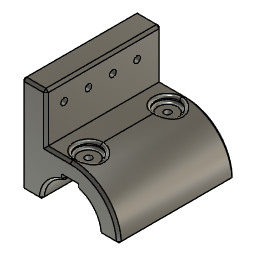
Assembly (Autodesk Fusion 360 archive; units mm, degrees)
design "motorbottlemount"
Autodesk Fusion 360 part; units mm, degrees
sketch "Sketch1" plane through (0, 0, 0) normal (0, 0, 1) x (1, 0, 0)
  line L0 (0, 0) -> (0, 65) construction
  circle A0 centre (0, 0) radius 2.7
  circle A1 centre (0, 65) radius 2.7
  dimension "d1" = 65
  dimension "d2" = 5.4
  dimension "d3" = 5.4
  constraint coincident L0.start A0.centre
  constraint vertical L0
  constraint coincident L0.end A1.centre
  measures "d1" distance of L0.start L0.end
  measures "d2" diameter of A0
  measures "d3" diameter of A1
sketch "Sketch2" plane through (0, 0, 0) normal (0, 1, 0) x (1, 0, 0)
  circle A0 centre (0, 0) radius 23.5
  circle A1 centre (0, 0) radius 40
  line L0 (-40, 0) -> (-40, -80)
  line L1 (-40, -80) -> (0, -80)
  line L2 (0, 0) -> (0, -80)
  line L3 (0, -80) -> (-20, -80)
  line L4 (-20, -80) -> (-20, -40)
  line L5 (-20, -40) -> (0, -40)
  line L6 (0, -40) -> (0, -80)
  line L7 (40, 0) -> (-40, 0)
  dimension "d4" = 47
  dimension "d5" = 80
  dimension "d6" = 80
  dimension "d8" = 20
  dimension "d9" = 40
  constraint coincident A0.centre A1.centre
  constraint concentric A0 A1
  constraint coincident A1 L0.start
  constraint tangent A1 L0
  constraint vertical L0
  constraint perpendicular L0 L1
  constraint coincident L1 L2.end
  constraint perpendicular L1 L2
  constraint horizontal L3
  constraint vertical L4
  constraint horizontal L5
  constraint midpoint L2 L5.end
  constraint coincident A1 L7.start
  constraint midpoint A0.centre L7
  measures "d4" diameter of A0
  measures "d5" diameter of A1
  measures "d6" distance of L0.start L0.end
  measures "d8" distance of L4.end L5.end
  measures "d9" distance of L3.end L4.end
extrude "Extrude1" add sketch "Sketch2" along normal blind 80 and the other way blind 15 contours A0 A1 L2 L7 | A0 A1 L2 L7 | A1 L0 L1 L4 L5
extrude "Extrude2" cut sketch "Sketch1" along normal blind 40
sketch "Sketch3" plane through (0, 0, 40) normal (0, 0, 1) x (-1, 0, 0)
  arc A0 (0, -67.7) -> (0, -62.3) centre (0, -65) ccw
  line L0 (0, -67.7) -> (0, -80)
  line L1 (0, -80) -> (20, -80)
  line L2 (20, -80) -> (20, 15)
  line L3 (20, 15) -> (0, 15)
  line L4 (0, 15) -> (0, 2.7)
  arc A1 (0, -2.7) -> (0, 2.7) centre (0, 0) ccw
  line L5 (0, -2.7) -> (0, -62.3)
  circle A2 centre (0, -65) radius 10
  circle A3 centre (0, 0) radius 10
  dimension "d16" = 20
  dimension "d17" = 20
  constraint concentric A0 A2
  constraint concentric A1 A3
  measures "d16" diameter of A2
  measures "d17" diameter of A3
extrude "Extrude3" cut sketch "Sketch3" against normal blind 5 contours A0 L0 L5 A2 | A0 L0 L5 A2 | L4 A1 L5 A3 | L4 A1 L5 A3
fillet "Fillet1" radius 2 6 edges at (-10, 65, 40) (10, 65, 38.7298) (-10, 0, 40) (10, 0, 38.7298) (9.3233, 61.3838, 35) (9.3233, -3.6162, 35)
sketch "Sketch4" plane through (-40, 0, 0) normal (-1, 0, 0) x (0, -1, 0)
  line L0 (15, 80) -> (-80, 80)
  line L1 (-80, 80) -> (-80, 0)
  line L2 (-80, 0) -> (15, 0)
  line L3 (15, 0) -> (15, 80)
  line L4 (15, 65) -> (13.1373, 65)
  line L5 (13.1373, 65) -> (-80, 65) construction
  circle A0 centre (0, 65) radius 2.7
  circle A1 centre (-20, 65) radius 2.7
  circle A2 centre (-40, 65) radius 2.7
  circle A3 centre (-60, 65) radius 2.7
  dimension "d22" = 15
  dimension "d23" = 5.4
  dimension "d24" = 15
  dimension "d27" = 60
  dimension "d28" = 0
  constraint coincident L3 L4.start
  constraint perpendicular L3 L4
  constraint coincident L1 L5.end
  constraint perpendicular L1 L5
  constraint coincident L5 A0.centre
  measures "d22" distance of L0 L5
  measures "d23" diameter of A0
  measures "d24" distance of L4.start A0.centre
extrude "Extrude4" cut sketch "Sketch4" against normal blind 30 contours A0 | A1 | A2 | A3
sketch "Sketch5" plane through (-40, 0, 0) normal (-1, 0, 0) x (0, -1, 0)
  circle A0 centre (-20, 65) radius 2.7
  circle A1 centre (-40, 65) radius 2.7
  circle A2 centre (0, 65) radius 2.7
  circle A3 centre (-60, 65) radius 2.7
  line L0 (15, 80) -> (-80, 80)
  line L1 (-80, 80) -> (-80, 0)
  line L2 (-80, 0) -> (15, 0)
  line L3 (15, 0) -> (15, 80)
  circle A4 centre (-60, 65) radius 7.5
  circle A5 centre (-40, 65) radius 7.5
  circle A6 centre (-20, 65) radius 7.5
  circle A7 centre (0, 65) radius 7.5
  dimension "d31" = 15
  dimension "d32" = 15
  dimension "d33" = 15
  dimension "d34" = 15
  constraint concentric A3 A4
  constraint concentric A1 A5
  constraint concentric A0 A6
  constraint concentric A2 A7
  measures "d31" diameter of A4
  measures "d32" diameter of A5
  measures "d33" diameter of A6
  measures "d34" diameter of A7
extrude "Extrude5" cut sketch "Sketch5" against normal blind 5 contours A4 | A5 | A6 | A7
sketch "Sketch6" plane through (0, -15, 0) normal (0, -1, 0) x (1, 0, 0)
  line L0 (-40, 0) -> (-23.5, 0)
  arc A0 (23.5, 0) -> (-23.5, 0) centre (0, 0) ccw
  line L1 (23.5, 0) -> (40, 0)
  arc A1 (40, 0) -> (0, 40) centre (0, 0) ccw
  line L2 (0, 40) -> (-20, 40)
  line L3 (-20, 40) -> (-20, 80)
  line L4 (-20, 80) -> (-40, 80)
  line L5 (-40, 80) -> (-40, 0)
  line L6 (5, 21.5) -> (-5, 21.5)
  line L7 (-5, 21.5) -> (-5, 25.5)
  line L8 (-5, 25.5) -> (5, 25.5)
  line L9 (5, 25.5) -> (5, 21.5)
  line L10 (5, 21.5) -> (-5, 25.5) construction
  line L11 (-5, 21.5) -> (5, 25.5) construction
  point P0 (0, 23.5)
  dimension "d40" = 10
  dimension "d41" = 4
  constraint horizontal L6
  constraint perpendicular L6 L7
  constraint parallel L6 L8
  constraint parallel L7 L9
  constraint coincident L10 P0
  constraint coincident L11 P0
  constraint midpoint A0 P0
  measures "d40" distance of L7.end L8.end
  measures "d41" distance of L6.end L7.end
extrude "Extrude6" cut sketch "Sketch6" against normal through all contours A0 L7 L8 L9
fillet "Fillet2" radius 2 8 edges at (-35, 66.9925, 67.7121) (-40, 66.9925, 67.7121) (-40, 46.9925, 67.7121) (-35, 46.9925, 67.7121) (-35, 26.9925, 67.7121) (-40, 26.9925, 67.7121) (-35, 6.9925, 67.7121) (-40, 6.9925, 67.7121)
chamfer "Chamfer1" distance 2 angle 45 2 edges at (-5, 32.5, 22.9619) (5, 32.5, 22.9619) 5 faces at (-34.5, 48.3333, 0) (34.5, 16.6667, 0) (-26.6667, 48.3333, 80) (-33.3333, 80, 40) (-33.3333, -15, 40)
